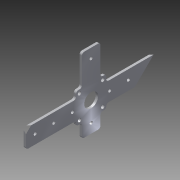
# Autodesk Inventor part: Plate
Saved by Autodesk Inventor 2014 (Build 180170000, 170)
## iProperties
Created: 2014-01-07
Part Number: Plate
Material: Aluminum 6061
Document SubType Name: Modeling
Designer: Andrew Toennies
Density: 2.71 g/cm^3
Appearance: Aluminum - Flat
Mass: 53.5982 g
Surface Area: 148.591 cm^2
Volume: 19.778 cm^3
Author: Andrew Toennies
Autodesk Inventor part; units mm, degrees
ref_plane "YZ Plane" through (0, 0, 0) normal (1, 0, 0) x (0, 1, 0)
ref_plane "XZ Plane" through (0, 0, 0) normal (0, 1, 0) x (-1, 0, 0)
ref_plane "XY Plane" through (0, 0, 0) normal (0, 0, 1) x (1, 0, 0)
sketch "Sketch1" plane through (0, 0, 0) normal (1, 0, 0) x (0, 1, 0)
  line L0 (101.6, 0) -> (101.6, -25.4)
  line L1 (0, -25.4) -> (0, 0)
  line L2 (101.6, -25.4) -> (60.2615, -25.4)
  line L3 (18.9865, 7.9375) -> (18.9865, 0)
  line L4 (18.9865, -25.4) -> (18.9865, -33.3375)
  line L5 (60.2615, 0) -> (101.6, 0)
  line L6 (60.2615, -33.3375) -> (60.2615, -25.4)
  line L7 (60.2615, 0) -> (60.2615, 7.9375)
  circle A0 centre (88.9, -12.7) radius 2.0828
  circle A1 centre (12.7, -12.7) radius 2.0828
  line L8 (55.499, 3.175) -> (23.749, 3.175) construction
  line L9 (23.749, 3.175) -> (23.749, -28.575) construction
  line L10 (23.749, -28.575) -> (55.499, -28.575) construction
  line L11 (55.499, -28.575) -> (55.499, 3.175) construction
  circle A2 centre (55.499, 3.175) radius 2.3876
  circle A3 centre (55.499, -28.575) radius 2.3876
  circle A4 centre (23.749, 3.175) radius 2.3876
  circle A5 centre (23.749, -28.575) radius 2.3876
  circle A6 centre (39.624, -12.7) radius 9.525
  line L12 (18.9865, 0) -> (0, 0)
  line L13 (0, -25.4) -> (18.9865, -25.4)
  line L14 (50.8, 7.9375) -> (50.8, 76.2)
  line L15 (50.8, 76.2) -> (25.4, 76.2)
  line L16 (25.4, 76.2) -> (25.4, 7.9375)
  line L17 (25.4, -33.3375) -> (25.4, -101.6)
  line L18 (25.4, -101.6) -> (50.8, -101.6)
  line L19 (50.8, -101.6) -> (50.8, -33.3375)
  line L20 (60.2615, 7.9375) -> (50.8, 7.9375)
  line L21 (25.4, 7.9375) -> (18.9865, 7.9375)
  line L22 (18.9865, -33.3375) -> (25.4, -33.3375)
  line L23 (50.8, -33.3375) -> (60.2615, -33.3375)
  circle A7 centre (38.1, 12.7) radius 2.0828
  circle A8 centre (38.1, -38.1) radius 2.0828
  circle A9 centre (38.1, 38.1) radius 2.0828
  circle A10 centre (38.1, 63.5) radius 2.0828
  circle A11 centre (38.1, -63.5) radius 2.0828
  circle A12 centre (38.1, -88.9) radius 2.0828
  dimension "d0" = 25.4
  dimension "d1" = 101.6
  dimension "d2" = 41.275
  dimension "d5" = 4.1656
  dimension "d6" = 4.1656
  dimension "d7" = 31.75
  dimension "d8" = 31.75
  dimension "d10" = 4.7625
  dimension "d11" = 12.7
  dimension "d12" = 12.7
  dimension "d13" = 12.7
  dimension "d15" = 4.7752
  dimension "d18" = 31.75
  dimension "d21" = 31.75
  dimension "d24" = 19.05
  dimension "d26" = 20.6375
  dimension "d29" = 61.976
  dimension "d31" = 12.7
  dimension "d32" = 25.4
  dimension "d33" = 25.4
  dimension "d34" = 76.2
  dimension "d35" = 25.4
  dimension "d36" = 76.2
  dimension "d40" = 41.275
  dimension "d41" = 4.7625
  dimension "d42" = 20.6375
  dimension "d44" = 4.1656
  dimension "d45" = 4.1656
  dimension "d46" = 12.7
  dimension "d47" = 12.7
  dimension "d50" = 25.4
  dimension "d55" = 12.7
  dimension "d56" = 12.7
  dimension "d59" = 25.4
  constraints: 48 end point, 16 parallel, 13 centre point, 12 perpendicular, 9 collinear, 5 horizontal, 3 vertical, 1 coincident, 14 other
  measures "d0" distance of L0.start L0.end
  measures "d1" distance of L0.end L1.start
  measures "d2" distance of L4.end L6.start
  measures "d5" diameter of A0
  measures "d6" diameter of A1
  measures "d7" distance of L10.end L8.start
  measures "d8" distance of L9.end L10.end
  measures "d10" distance between parallel lines of L7 L11
  measures "d11" distance from line of L0 A0.centre
  measures "d12" distance from line of L2 A0.centre
  measures "d13" distance from line of A1.centre L1
  measures "d15" diameter of A2
  measures "d18" distance of A2.centre A3.centre
  measures "d21" distance of A2.centre A4.centre
  measures "d24" diameter of A6
  measures "d26" distance from line of L7 A6.centre
  measures "d29" distance from line of L0 A6.centre
  measures "d31" distance from line of L12 A1.centre
  measures "d32" distance of L14.end L15.end
  measures "d33" distance between parallel lines of L16 L1
  measures "d34" distance between parallel lines of L12 L15
  measures "d35" distance of L17.end L18.end
  measures "d36" distance between parallel lines of L18 L13
  measures "d40" distance between parallel lines of L21 L22
  measures "d41" distance between parallel lines of L23 L10
  measures "d42" distance from line of L23 A6.centre
  measures "d44" diameter of A7
  measures "d45" diameter of A8
  measures "d46" distance from line of L14 A7.centre
  measures "d47" distance from line of L12 A7.centre
  measures "d50" distance of A7.centre A9.centre
  measures "d55" distance from line of L19 A8.centre
  measures "d56" distance from line of A8.centre L2
  measures "d59" distance of A8.centre A11.centre
extrude "Extrusion1" add sketch "Sketch1" along normal blind 3.175
sketch "Sketch2" plane through (3.175, 0, 0) normal (1, 0, 0) x (0, 0, -1)
  circle A0 centre (88.9, 38.1) radius 2.0828 projected
  circle A1 centre (63.5, 38.1) radius 2.0828 projected
  circle A2 centre (-63.5, 38.1) radius 2.0828 projected
  circle A3 centre (-38.1, 38.1) radius 2.0828 projected
  circle A4 centre (88.9, 38.1) radius 4.7625
  circle A5 centre (63.5, 38.1) radius 4.7625
  circle A6 centre (-38.1, 38.1) radius 4.7625
  circle A7 centre (-63.5, 38.1) radius 4.7625
  dimension "d64" = 9.525
  dimension "d65" = 9.525
  dimension "d66" = 9.525
  dimension "d67" = 9.525
  constraints: 4 centre point, 4 coincident
  measures "d64" diameter of A4
  measures "d65" diameter of A5
  measures "d66" diameter of A6
  measures "d67" diameter of A7
extrude "Extrusion2" cut sketch "Sketch2" against normal blind 25.4 contours A0 | A1 | A4 | A5 | A6 | A7
body "Solid1"
